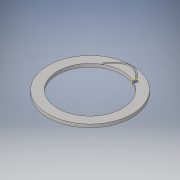
# Autodesk Inventor part: NewCam02
Saved by Autodesk Inventor 2016 (Build 200138000, 138)
## iProperties
Created: 2015-07-23
Part Number: NewCam02
Material: Generic
Document SubType Name: Modeling
Designer: steele
Density: 1 g/cm^3
Appearance: Default
Author: steele
Autodesk Inventor part; units mm, degrees
ref_plane "YZ Plane" through (0, 0, 0) normal (1, 0, 0) x (0, 1, 0)
ref_plane "XZ Plane" through (0, 0, 0) normal (0, 1, 0) x (-1, 0, 0)
ref_plane "XY Plane" through (0, 0, 0) normal (0, 0, 1) x (1, 0, 0)
sketch "Sketch1" plane through (0, 0, 0) normal (0, 1, 0) x (-1, 0, 0)
  circle A0 centre (0, 0) radius 127
  circle A1 centre (0, 0) radius 165.1
  dimension "innerDiameter" = 254
  dimension "outerDiameter" = 330.2
  constraints: 2 centre point, 2 coincident
  measures "innerDiameter" diameter of A0
  measures "outerDiameter" diameter of A1
extrude "Extrusion1" add sketch "Sketch1" against normal blind 12.7
sketch "Sketch2" plane through (0, 0, 0) normal (0, 1, 0) x (1, 0, 0)
  circle A0 centre (0, 0) radius 130.175 construction
  circle A1 centre (0, 0) radius 161.925 construction
  line L0 (0, 0) -> (0, 161.925) construction
  line L1 (0, 0) -> (80.9625, 140.2312) construction
  line L2 (0, 0) -> (-80.9625, 140.2312) construction
  line L3 (65.0875, 112.7349) -> (0, 210.2928) construction
  line L4 (0, 210.2928) -> (-65.0875, 112.7349) construction
  spline S0 degree 2 poles (65.0875, 112.7349) (0, 210.2928) (-65.0875, 112.7349) knots 1 1 1 2 2 2
  dimension "d4" = 260.35
  dimension "d5" = 323.85
  dimension "arcForCam" = 30
  dimension "d7" = 30
  constraints: 6 end point, 5 point on circle, 3 point on line, 2 centre point, 2 coincident, 1 vertical, 3 other
  measures "d4" diameter of A0
  measures "d5" diameter of A1
  measures "arcForCam" angle of L0 L1
  measures "d7" angle of L2 L0
ref_plane "Work Plane2" through (65.0875, 0, -112.7349) normal (-0.5549886, 0, -0.831858) x (0, -1, 0)
sketch "Sketch4" plane through (65.0875, 0, -112.7349) normal (-0.5549886, 0, -0.831858) x (0, -1, 0)
  circle A0 centre (0, 0) radius 2.7908
  point P0 (0, 116.7101)
  constraints: 1 centre point
sweep "Sweep1" cut profiles "Sketch4" path "Sketch2"
equation "\"d7\" = arcForCam"
body "Solid1"
